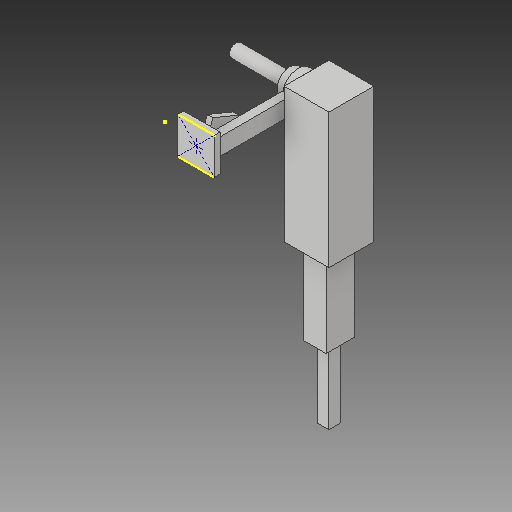
# Autodesk Inventor part: simp_burnisher
Saved by Autodesk Inventor 2019 (Build 230136000, 136)
## iProperties
Created: 2019-11-07
Part Number: simp_burnisher
Material: Generic
Document SubType Name: Modeling
Designer: luua
Density: 1 g/cm^3
Appearance: Default
Author: luua
Autodesk Inventor part; units mm, degrees
ref_plane "YZ Plane" through (0, 0, 0) normal (1, 0, 0) x (0, 1, 0)
ref_plane "XZ Plane" through (0, 0, 0) normal (0, 1, 0) x (-1, 0, 0)
ref_plane "XY Plane" through (0, 0, 0) normal (0, 0, 1) x (1, 0, 0)
sketch "Sketch1" plane through (0, 0, 0) normal (0, 0, 1) x (1, 0, 0)
  line L0 (-76.6085, 0) -> (76.6085, 0) construction
  line L1 (-48, 0) -> (48, 0)
  line L2 (48, 0) -> (48, 11)
  line L3 (48, 11) -> (-48, 11)
  line L4 (-48, 11) -> (-48, 0)
  point P0 (0, 0)
  point P1 (0, 0)
  point P2 (0, 11)
  dimension "d0" = 96
  dimension "d1" = 11
  constraints: 10 end point, 2 horizontal, 2 midpoint, 2 parallel, 1 coincident, 1 perpendicular, 1 point on line, 1 vertical alignment
  measures "d0" distance of L2.end L3.end
  measures "d1" distance of L1.end L2.end
revolve "Revolution1" add sketch "Sketch1" angle 360 about axis through (-76.6085, 0, 0) along (1, 0, 0)
sketch "Sketch2" plane through (48, 0, 0) normal (1, 0, 0) x (0, 0, -1)
  circle A0 centre (0, 0) radius 22.5
  dimension "d3" = 45
  constraints: 1 centre point, 1 coincident
  measures "d3" diameter of A0
extrude "Extrusion1" add sketch "Sketch2" along normal blind 30
sketch "Sketch3" plane through (0, 0, 0) normal (0, 0, 1) x (1, 0, 0)
  line L0 (78, -22.5) -> (78, 22.5) projected
  line L1 (78, 27.5) -> (78, -212.5)
  line L2 (48, 22.5) -> (78, 22.5) projected
  line L3 (48, -22.5) -> (78, -22.5) projected
  line L4 (78, 27.5) -> (158, 27.5)
  line L5 (158, 27.5) -> (158, -212.5)
  line L6 (78, -212.5) -> (98, -212.5)
  line L7 (158, -212.5) -> (138, -212.5)
  line L8 (118, 27.5) -> (118, -212.5) construction
  line L9 (98, -212.5) -> (98, -362.5)
  line L10 (98, -362.5) -> (138, -362.5)
  line L11 (138, -362.5) -> (138, -212.5)
  line L12 (108, -362.5) -> (128, -362.5)
  line L13 (128, -362.5) -> (128, -492.5)
  line L14 (128, -492.5) -> (108, -492.5)
  line L15 (108, -492.5) -> (108, -362.5)
  line L16 (138, -212.5) -> (98, -212.5)
  point P0 (0, 0)
  point P1 (118, -362.5)
  dimension "d6" = 5
  dimension "d7" = 190
  dimension "d8" = 80
  dimension "d9" = 40
  dimension "d10" = 150
  dimension "d36" = 20
  dimension "d37" = 130
  constraints: 28 end point, 6 horizontal, 3 midpoint, 3 perpendicular, 3 vertical, 2 collinear, 2 parallel, 1 horizontal alignment, 1 symmetric about line
  measures "d6" distance from line of L1.start L2
  measures "d7" distance from line of L1.end L3
  measures "d8" distance of L1.start L4.end
  measures "d9" distance of L6.end L7.end
  measures "d10" distance of L6.end L9.end
  measures "d36" distance of L13.end L14.end
  measures "d37" distance of L12.end L13.end
extrude "Extrusion2" add sketch "Sketch3" along normal mid plane 80 contours L0 L1 L4 L5 L7 L16 L6
sketch "Sketch4" plane through (78, -212.5, 40) normal (-1, 0, 0) x (0, 0, 1)
  circle A0 centre (-40, 212.5) radius 22.5 projected
  circle A1 centre (-40, 212.5) radius 27.5
  line L0 (-13.229, 218.7899) -> (123.9314, 218.7899)
  line L1 (123.9314, 218.7899) -> (123.9314, 188.7899)
  line L2 (123.9314, 188.7899) -> (-26.0686, 188.7899)
  line L3 (0, 240) -> (0, 0) projected
  dimension "d13" = 55
  dimension "d14" = 150
  dimension "d15" = 90
  dimension "d16" = 30
  dimension "d17" = 90
  constraints: 6 end point, 2 point on circle, 1 centre point, 1 coincident, 1 perpendicular
  measures "d13" diameter of A1
  measures "d14" distance of L1.end L2.end
  measures "d15" angle of L1 L2
  measures "d16" distance of L0.end L1.end
  measures "d17" angle of L3 L2
extrude "Extrusion3" add sketch "Sketch4" along normal blind 15
extrude "Extrusion7" add sketch "Sketch3" along normal mid plane 50 contours L16 L11 L10 L9
extrude "Extrusion8" add sketch "Sketch3" along normal mid plane 20 contours L10 L13 L14 L15
sketch "Sketch5" plane through (63, -212.5, 40) normal (-1, 0, 0) x (0, 0, 1)
  line L0 (123.9314, 218.7899) -> (-13.229, 218.7899) projected
  circle A0 centre (-40, 212.5) radius 22.5 projected
  arc A1 (-13.229, 218.7899) -> (-26.0686, 188.7899) centre (-40, 212.5) ccw projected
  line L1 (-26.0686, 188.7899) -> (123.9314, 188.7899) projected
  line L2 (123.9314, 188.7899) -> (123.9314, 218.7899) projected
  line L3 (123.9314, 218.7899) -> (-13.229, 218.7899) projected
  line L4 (123.9314, 188.7899) -> (123.9314, 218.7899) projected
  line L5 (131.903, 190.2883) -> (111.482, 239.6833)
  line L6 (111.482, 239.6833) -> (65.2751, 220.5803)
  line L7 (65.2751, 220.5803) -> (85.6962, 171.1852)
  line L8 (131.903, 190.2883) -> (85.6962, 171.1852)
  point P0 (123.9314, 203.7899)
  dimension "d61" = 50
  constraints: 8 end point, 2 perpendicular, 1 midpoint, 1 parallel
  measures "d61" distance of L6.end L5.end
sketch "Sketch9" plane through (78, -23.7101, 163.9314) normal (0, 0, 1) x (1, 0, 0)
  line L0 (0, 0) -> (0, 30) projected
  line L1 (9.9045, 47.5) -> (-55.0955, 47.5)
  line L2 (-55.0955, 47.5) -> (-55.0955, -17.5)
  line L3 (-55.0955, -17.5) -> (9.9045, -17.5)
  line L4 (9.9045, -17.5) -> (9.9045, 47.5)
  line L5 (25, 47.5) -> (-40, -17.5) construction
  line L6 (-40, 47.5) -> (25, -17.5) construction
  point P0 (-78, 23.7101)
  dimension "d56" = 65
  dimension "d57" = 65
  constraints: 12 end point, 2 parallel, 1 horizontal, 1 perpendicular
  measures "d56" distance of L3.end L2.end
  measures "d57" distance of L2.end L1.end
extrude "Extrusion10" add sketch "Sketch9" along normal blind 10 separate body
extrude "Extrusion11" add sketch "Sketch5" along normal blind 10 contours L5 L2 L1 L7 L0 | L0 L7 L6 L5 | L5 L8 L7 L1 L2 bodies 1
sketch "Sketch10" plane through (78, -23.7101, 173.9314) normal (0, 0, 1) x (1, 0, 0)
  line L0 (-55.0955, -17.5) -> (9.9045, -17.5) projected
  line L1 (9.9045, 47.5) -> (-55.0955, 47.5) projected
  line L2 (9.9045, -17.5) -> (-55.0955, 47.5) construction
  line L3 (9.9045, 47.5) -> (-55.0955, -17.5) construction
  point P0 (-78, 23.7101)
  point P1 (-22.5955, 15)
  constraints: 4 end point, 1 midpoint
body "Solid1"
body "Solid2"
